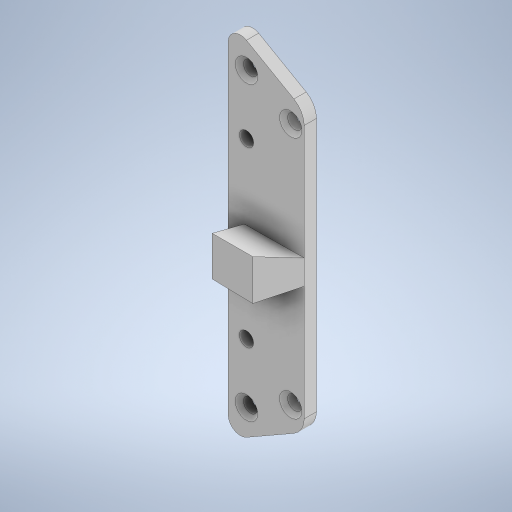
# Autodesk Inventor part: AcopleCamara-part1
Saved by Autodesk Inventor 2023 (Build 270158000, 158)
## iProperties
Created: 2023-12-18
Part Number: AcopleCamara-part1
Material: Genérico
Document SubType Name: Modeling
Designer: ASUS
Density: 1 g/cm^3
Appearance: Valor por defecto
Author: ASUS
Autodesk Inventor part; units mm, degrees
ref_plane "YZ Plane" through (0, 0, 0) normal (1, 0, 0) x (0, 1, 0)
ref_plane "XZ Plane" through (0, 0, 0) normal (0, 1, 0) x (-1, 0, 0)
sketch "Boceto1" plane through (0, 0, 0) normal (0, 0, 1) x (1, 0, 0)
  line L0 (134.9, 24.045) -> (134.9, 29.745)
  arc A0 (134.9, 24.045) -> (137.5, 24.045) centre (136.2, 24.045) ccw
  line L1 (137.5, 29.745) -> (137.5, 24.045)
  circle A1 centre (136.2, 29.745) radius 1.3 construction
  line L2 (126.9, 35.7) -> (126.9, 21.2)
  line L3 (123.9, 21.2) -> (123.9, 35.7)
  circle A2 centre (125.4, 35.7) radius 1.5 construction
  circle A3 centre (125.4, 21.2) radius 1.5 construction
  line L4 (126.8891, -21.2025) -> (126.8816, -35.7004)
  circle A4 centre (125.3854, -21.2022) radius 1.5037 construction
  line L5 (123.8816, -35.6996) -> (123.8816, -21.2019)
  circle A5 centre (125.3816, -35.6996) radius 1.5 construction
  circle A6 centre (136.1847, -29.7501) radius 1.3 construction
  line L6 (137.4876, -24.0508) -> (137.4847, -29.7508)
  arc A7 (137.4876, -24.0508) -> (134.8876, -24.0494) centre (136.1876, -24.0501) ccw
  line L7 (134.8847, -29.7494) -> (134.8876, -24.0494)
  line L8 (120.8816, 55.9985) -> (120.8816, -0.0015)
  line L9 (139.5, 56.008) -> (139.5, -0.0015)
  line L10 (50.0101, -56.038) -> (139.5, -55.992)
  line L11 (139.5, 56.008) -> (49.9528, 55.962)
  line L12 (136.8302, -30.8785) -> (126.1265, -37.0016) construction
  line L13 (136.9827, -35.3995) -> (125.3713, -42.0418)
  arc A8 (192.3943, -3.7013) -> (191.4002, 0.0347) centre (191.4012, -1.9653) ccw
  line L14 (120.8816, -0.0015) -> (120.8816, -39.4378)
  line L15 (139.5, -0.0015) -> (139.5, -31.0595)
  arc A9 (120.8816, -39.4378) -> (125.3713, -42.0418) centre (123.8816, -39.4378) ccw
  arc A10 (136.9827, -35.3995) -> (139.5, -31.0595) centre (134.5, -31.0595) ccw
  line L16 (139.5, -0.0015) -> (120.8816, -0.0015) construction
  line L17 (136.9827, 35.3964) -> (125.3713, 42.0388)
  arc A11 (125.3713, 42.0388) -> (120.8816, 39.4347) centre (123.8816, 39.4347) ccw
  arc A12 (139.5, 31.0564) -> (136.9827, 35.3964) centre (134.5, 31.0564) ccw
  line L18 (137.2847, -29.7507) -> (137.2876, -24.0507)
  arc A13 (137.2876, -24.0507) -> (135.0876, -24.0495) centre (136.1876, -24.0501) ccw
  line L19 (135.0876, -24.0495) -> (135.0847, -29.7495)
  arc A14 (135.0847, -29.7495) -> (137.2847, -29.7507) centre (136.1847, -29.7501) ccw
  line L20 (126.6816, -35.7003) -> (126.6891, -21.2024)
  arc A15 (126.6891, -21.2024) -> (124.0816, -21.2022) centre (125.3854, -21.2022) ccw
  line L21 (124.0816, -21.2022) -> (124.0816, -35.6996)
  arc A16 (124.0816, -35.6996) -> (126.6816, -35.7003) centre (125.3816, -35.6996) ccw
  arc A17 (135.1, 24.045) -> (137.3, 24.045) centre (136.2, 24.045) ccw
  line L22 (135.1, 24.045) -> (135.1, 29.745)
  arc A18 (137.3, 29.745) -> (135.1, 29.745) centre (136.2, 29.745) ccw
  line L23 (137.3, 29.745) -> (137.3, 24.045)
  line L24 (126.7, 21.2) -> (126.7, 35.7)
  arc A19 (126.7, 35.7) -> (124.1, 35.7) centre (125.4, 35.7) ccw
  line L25 (124.1, 35.7) -> (124.1, 21.2)
  arc A20 (124.1, 21.2) -> (126.7, 21.2) centre (125.4, 21.2) ccw
  circle A21 centre (125.3816, -35.6996) radius 1.75
  circle A22 centre (136.1847, -29.7501) radius 1.75
  circle A23 centre (125.4, 35.7) radius 1.75
  circle A24 centre (136.2, 29.745) radius 1.75
  circle A25 centre (125.4, 21.2) radius 1.75
  circle A26 centre (125.3854, -21.2022) radius 1.75
  point P0 (0, 0)
  point P1 (120.8816, -56.0015)
  point P2 (139.5, -33.9595)
  point P3 (120.8816, -44.6101)
  point P4 (126.7, 34.5285)
  point P5 (124.1, 34.5285)
  point P6 (137.3, 28.3839)
  point P7 (135.1, 28.3839)
  point P8 (124.0816, -34.5281)
  point P9 (126.6823, -34.5287)
  point P10 (135.0854, -28.3885)
  point P11 (137.2854, -28.3896)
  dimension "d0" = 3
  dimension "d1" = 2
  dimension "d2" = 4
  dimension "d3" = 2
  dimension "d4" = 3
  dimension "d5" = 5
  dimension "d8" = 0.2
  dimension "d9" = 0.2
  dimension "d10" = 0.2
  dimension "d11" = 0.2
  dimension "d14" = 3.5
  dimension "d15" = 3.5
  dimension "d16" = 3.5
  dimension "d17" = 3.5
  dimension "d18" = 3.5
  dimension "d19" = 3.5
  constraints: 52 end point, 44 point on circle, 27 centre point, 11 point on line, 7 tangent, 6 coincident, 4 symmetric about line, 2 vertical, 1 horizontal, 1 parallel, 6 other
  measures "d0" distance between parallel lines of L5 L8
  measures "d1" distance between parallel lines of L1 L9
  measures "d2" distance between parallel lines of L12 L13
  measures "d3" radius of A8
  measures "d4" radius of A9
  measures "d5" radius of A10
  measures "d8" distance between parallel lines of L6 L18
  measures "d9" distance between parallel lines of L4 L20
  measures "d10" distance between parallel lines of L1 L23
  measures "d11" distance between parallel lines of L2 L24
  measures "d14" diameter of A21
  measures "d15" diameter of A22
  measures "d16" diameter of A23
  measures "d17" diameter of A24
  measures "d18" diameter of A25
  measures "d19" diameter of A26
extrude "Extrusión1" add sketch "Boceto1" along normal blind 3 contours L0 A24 L22 A17 L23 L1 A0 | A24 L23 A18 L22 | A24 L23 A17 L22 | L22 A18 L23 A24 | L2 A25 L24 A23 | A23 L24 A19 L25 | A23 L25 A19 L24 | L24 A25 L25 A23 | L25 A25 L3 A23 | L4 A21 L20 A26 | A21 L21 A16 L20 | L20 A21 L21 A26 | L20 A16 L21 A21 | L21 A21 L5 A26 | L6 A22 L18 A13 L19 L7 A7 | A22 L19 A14 L18 | A22 L19 A13 L18 | L18 A14 L19 A22 | A11 L17 A12 L9 L15 A10 L13 A9 L14 L8
extrude "Extrusión2" [suppressed]
sketch "Boceto2" plane through (0, 0, 3) normal (0, 0, 1) x (1, 0, 0)
  point P0 (0, 0)
  point P1 (125.4, 35.7)
  point P2 (136.2, 29.745)
  point P3 (125.4, 21.2)
  point P4 (136.1847, -29.7501)
  point P5 (125.3854, -21.2022)
  point P6 (125.3816, -35.6996)
hole "Agujero1" at (125.4, 35.7, 3) at (136.2, 29.745, 3) at (136.1847, -29.7501, 3) at (125.3816, -35.6996, 3) direction (0, 0, -1) diameter 3.5 end through all countersink diameter 5.5 countersink angle 90
ref_plane "Plano de trabajo1" through (130.1908, -31.0595, 0) normal (1, 0, 0) x (0, 0, -1)
sketch "Boceto3" plane through (139.5, -31.0595, 0) normal (1, 0, 0) x (0, 0, -1)
  line L0 (-3, 31.0579) -> (-11, 31.0579) construction
  line L1 (-11, 26.0579) -> (-11, 36.0579)
  line L2 (-11, 26.0579) -> (-3, 28.0579)
  line L3 (-11, 36.0579) -> (-3, 34.0579)
  line L4 (0, 0) -> (0, 62.1159)
  line L5 (-3, 28.0579) -> (0, 28.0579)
  line L6 (-3, 34.0579) -> (0, 34.0579)
  line L7 (-3, 0) -> (-3, 28.0579)
  line L8 (-3, 34.0579) -> (-3, 62.1159)
  line L9 (-3, 0) -> (-3, 28.0579)
  line L10 (-3, 34.0579) -> (-3, 62.1159)
  point P0 (0, 31.0595)
  dimension "d27" = 8
  dimension "d28" = 10
  dimension "d29" = 6
  constraints: 22 end point, 2 horizontal, 2 point on line, 1 midpoint, 1 perpendicular, 1 vertical
  measures "d27" distance of L0.end L0.start
  measures "d28" distance of L1.start L1.end
  measures "d29" distance of L2.end L3.end
extrude "Extrusión3" add sketch "Boceto3" against normal blind 14.618 draft -0.5
sketch "Boceto4" plane through (0, 0, 0) normal (0, 1, 0) x (-1, 0, 0)
  line L0 (-124.882, 10.8724) -> (-124.882, 3.0157) projected
  line L1 (-139.5, 3) -> (-124.882, 3.0157) projected
  line L2 (-139.5, 11) -> (-139.5, 3) projected
  line L3 (-139.5, 11) -> (-124.882, 10.8724) projected
  line L4 (-139.5, 3) -> (-134.9044, 10.9599)
  point P0 (0, 0)
  dimension "d32" = 30
  constraints: 2 end point, 1 point on line
  measures "d32" angle of L2 L4
extrude "Extrusión4" cut sketch "Boceto4" along normal through all both and the other way through all contours L4 L2 L3
